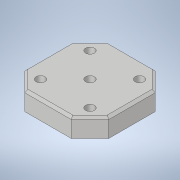
# Autodesk Inventor part: Platform A
Saved by Autodesk Inventor 2022 (Build 260153000, 153)
## iProperties
Created: 2021-01-07
Part Number: Platform A
Material: Generic
Document SubType Name: Modeling
Designer: caleb
Density: 1 g/cm^3
Appearance: Default
Author: caleb
Autodesk Inventor part; units mm, degrees
ref_plane "YZ Plane" through (0, 0, 0) normal (1, 0, 0) x (0, 1, 0)
ref_plane "XZ Plane" through (0, 0, 0) normal (0, 1, 0) x (-1, 0, 0)
ref_plane "XY Plane" through (0, 0, 0) normal (0, 0, 1) x (1, 0, 0)
sketch "Sketch1" plane through (0, 0, 0) normal (0, 1, 0) x (-1, 0, 0)
  line L0 (-14.2875, 14.2875) -> (14.2875, 14.2875)
  line L1 (14.2875, 14.2875) -> (14.2875, -14.2875)
  line L2 (14.2875, -14.2875) -> (-14.2875, -14.2875)
  line L3 (-14.2875, -14.2875) -> (-14.2875, 14.2875)
  line L4 (-14.2875, 14.2875) -> (14.2875, -14.2875) construction
  line L5 (14.2875, 14.2875) -> (-14.2875, -14.2875) construction
  point P0 (0, 0)
  dimension "d0" = 28.575
  dimension "d1" = 28.575
  constraints: 12 end point, 2 midpoint, 2 parallel, 1 horizontal, 1 perpendicular
  measures "d0" distance of L0.end L1.end
  measures "d1" distance of L0.start L0.end
extrude "Extrusion1" add sketch "Sketch1" along normal blind 6.35
sketch "Sketch2" plane through (0, 6.35, 0) normal (0, 1, 0) x (1, 0, 0)
  circle A0 centre (-8.4201, -8.4201) radius 1.4986
  line L0 (-14.2875, 14.2875) -> (-14.2875, -14.2875) projected
  line L1 (-14.2875, -14.2875) -> (14.2875, -14.2875) projected
  circle A1 centre (-8.4201, 8.4201) radius 1.4986
  circle A2 centre (8.4201, -8.4201) radius 1.4986
  circle A3 centre (8.4201, 8.4201) radius 1.4986
  point P0 (0, 0)
  dimension "d4" = 2.9972
  dimension "d5" = 8.4201
  dimension "d8" = 16.8402
  dimension "d11" = 16.8402
  dimension "d14" = 8.4201
  constraints: 4 centre point, 1 horizontal, 1 vertical, 6 other
  measures "d4" diameter of A0
  measures "d5" horizontal distance of A0.centre point (0, 0)
  measures "d8" distance of A0.centre A1.centre
  measures "d11" distance of A0.centre A2.centre
  measures "d14" horizontal distance of point (0, 0) A0.centre
hole "Hole1" at (8.4201, 6.35, -8.4201) at (-8.4201, 6.35, -8.4201) at (-8.4201, 6.35, 8.4201) at (8.4201, 6.35, 8.4201) direction (0, -1, 0) diameter 2.9972 end through all
sketch "Sketch3" plane through (0, 6.35, 0) normal (0, 1, 0) x (1, 0, 0)
  circle A0 centre (0, 0) radius 1.4986
  dimension "d22" = 2.9972
  constraints: 1 centre point, 1 coincident
  measures "d22" diameter of A0
extrude "Extrusion2" cut sketch "Sketch3" against normal through all
sketch "Sketch4" plane through (0, 0, 0) normal (0, -1, 0) x (1, 0, 0)
  line L0 (-6.33, -1.2362) -> (2.4965, -8.3482)
  line L1 (5.08, -7.112) -> (5.08, 7.112)
  line L2 (2.4965, 8.3482) -> (-6.33, 1.2362)
  arc A0 (5.08, 7.112) -> (2.4965, 8.3482) centre (3.4925, 7.112) ccw
  arc A1 (-6.33, 1.2362) -> (-6.33, -1.2362) centre (-5.334, 0) ccw
  arc A2 (2.4965, -8.3482) -> (5.08, -7.112) centre (3.4925, -7.112) ccw
  circle A3 centre (0, 0) radius 1.4986 projected
  dimension "d42" = 1.5875
  dimension "d43" = 14.224
  dimension "d44" = 7.112
  dimension "d45" = 5.334
  dimension "d46" = 5.08
  constraints: 6 end point, 6 point on circle, 6 tangent, 3 centre point, 2 equal radius, 1 horizontal alignment, 1 vertical
  measures "d42" radius of A0
  measures "d43" distance of A0.centre A2.centre
  measures "d44" vertical distance of A0.centre A3.centre
  measures "d45" distance of A3.centre A1.centre
  measures "d46" distance from line of L1 A3.centre
extrude "Extrusion3" cut sketch "Sketch4" against normal blind 1.4986
chamfer "Chamfer3" distance 6.35 angle 45 4 edges at (14.2875, 3.175, -14.2875) (-14.2875, 3.175, -14.2875) (-14.2875, 3.175, 14.2875) (14.2875, 3.175, 14.2875)
chamfer "Chamfer4" distance 0.7937 angle 45 8 edges at (11.1125, 6.35, -11.1125) (0, 6.35, -14.2875) (-11.1125, 6.35, -11.1125) (-14.2875, 6.35, 0) (-11.1125, 6.35, 11.1125) (0, 6.35, 14.2875) (11.1125, 6.35, 11.1125) (14.2875, 6.35, 0)
equation "\"d44\" = 0.5 * d43"
body "Solid1"
